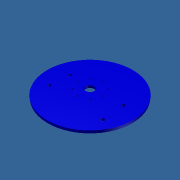
# Autodesk Inventor part: Acrylic_rotationServoTray
Saved by Autodesk Inventor 2012 (Build 160160000, 160)
## iProperties
Created: 2014-03-29
Part Number: Acrylic_rotationServoTray
Material: Default
Document SubType Name: Modeling
Designer: Admin
Density: 1 g/cm^3
Author: Admin
Autodesk Inventor part; units mm, degrees
ref_plane "YZ Plane" through (0, 0, 0) normal (1, 0, 0) x (0, 1, 0)
ref_plane "XZ Plane" through (0, 0, 0) normal (0, 1, 0) x (-1, 0, 0)
ref_plane "XY Plane" through (0, 0, 0) normal (0, 0, 1) x (1, 0, 0)
sketch "Sketch1" plane through (0, 0, 0) normal (0, 0, 1) x (1, 0, 0)
  circle A0 centre (0, 0) radius 50
  dimension "d0" = 100
  constraints: 1 centre point, 1 coincident
  measures "d0" diameter of A0
extrude "Extrusion1" add sketch "Sketch1" along normal blind 2.8
sketch "Sketch2" plane through (0, 0, 2.8) normal (0, 0, 1) x (1, 0, 0)
  circle A0 centre (0, 0) radius 50 projected
  circle A1 centre (0, 0) radius 5
  dimension "d3" = 10
  constraints: 1 centre point, 1 coincident
  measures "d3" diameter of A1
extrude "Extrusion2" cut sketch "Sketch2" against normal through all contours A1
sketch "Sketch3" plane through (0, 0, 2.8) normal (0, 0, 1) x (1, 0, 0)
  circle A0 centre (0, 0) radius 5 projected
  line L0 (-70, 0) -> (70, 0) projected
  line L1 (0, -70) -> (0, 70) projected
  circle A1 centre (0, 14.84) radius 1
  circle A2 centre (-10.4935, 10.4935) radius 1
  circle A3 centre (-14.84, 0) radius 1
  circle A4 centre (-10.4935, -10.4935) radius 1
  circle A5 centre (0, -14.84) radius 1
  circle A6 centre (10.4935, -10.4935) radius 1
  circle A7 centre (14.84, 0) radius 1
  circle A8 centre (10.4935, 10.4935) radius 1
  circle A9 centre (-28, 2.3) radius 1.825
  circle A10 centre (-28, -21.1) radius 1.825
  circle A11 centre (33.8, -21.1) radius 1.825
  circle A12 centre (33.8, 2.3) radius 1.825
  dimension "d6" = 2
  dimension "d7" = 14.84
  dimension "d10" = 360
  constraints: 12 centre point, 1 point on line, 25 other
  measures "d6" diameter of A1
  measures "d7" distance from line of A1.centre L0
extrude "Extrusion3" cut sketch "Sketch3" against normal through all contours A5 L1 | L1 A5 | A3 L0 | L0 A3 | A1 L1 | L1 A1 | A7 L0 | L0 A7 | A2 | A4 | A6 | A8 | A9 | A10 | A11 | A12
body "Solid1"
